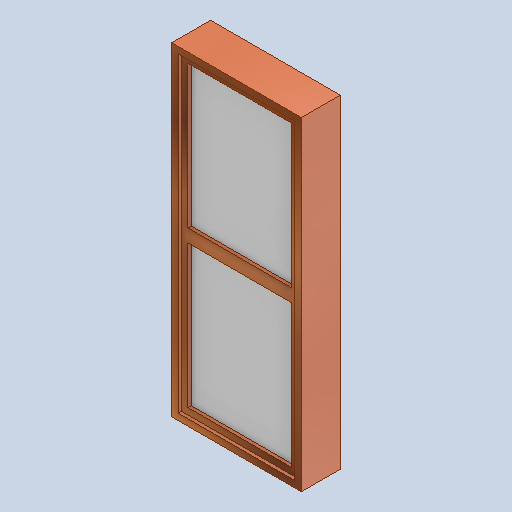
# Autodesk Inventor part: 窗_無底
Saved by Autodesk Inventor 2024.2 (Build 282272000, 272)
## iProperties
Created: 2024-05-31
Part Number: 窗_無底
Material: 木材 (胡桃木)
Document SubType Name: Modeling
Designer: User
Density: 0.55 g/cm^3
Appearance: 胡桃木 - 天然拋光
Author: User
Autodesk Inventor part; units mm, degrees
ref_plane "YZ Plane" through (0, 0, 0) normal (1, 0, 0) x (0, 1, 0)
ref_plane "XZ Plane" through (0, 0, 0) normal (0, 1, 0) x (-1, 0, 0)
ref_plane "XY Plane" through (0, 0, 0) normal (0, 0, 1) x (1, 0, 0)
sketch "草圖1" plane through (0, 0, 0) normal (0, 0, 1) x (1, 0, 0)
  line L0 (-1, 2.5) -> (1, 2.5)
  line L1 (1, 2.5) -> (1, -2.5)
  line L2 (1, -2.5) -> (-1, -2.5)
  line L3 (-1, -2.5) -> (-1, 2.5)
  line L4 (-1, 2.5) -> (1, -2.5) construction
  line L5 (1, 2.5) -> (-1, -2.5) construction
  line L6 (-0.8, -0.1) -> (0.8, -0.1)
  line L7 (1, -0.1) -> (1, 0.1)
  line L8 (0.8, 0.1) -> (-0.8, 0.1)
  line L9 (-1, 0.1) -> (-1, -0.1)
  line L10 (-1, -0.1) -> (1, 0.1) construction
  line L11 (1, -0.1) -> (-1, 0.1) construction
  line L12 (-0.8, -2.3) -> (0.8, -2.3)
  line L13 (0.8, 2.3) -> (-0.8, 2.3)
  line L14 (-0.8, 2.3) -> (0.8, -2.3) construction
  line L15 (-0.8, -2.3) -> (0.8, 2.3) construction
  line L16 (0.8, -2.3) -> (0.8, -0.08)
  line L17 (0.8, 0.08) -> (0.8, 2.3)
  line L18 (-0.8, 2.3) -> (-0.8, 0.08)
  line L19 (-0.8, -0.08) -> (-0.8, -2.3)
  line L20 (-1, -2.5) -> (1, -2.5)
  line L21 (1, -2.5) -> (1, -5.5)
  line L22 (1, -5.5) -> (-1, -5.5)
  line L23 (-1, -5.5) -> (-1, -2.5)
  line L24 (-0.9, -2.4) -> (0.9, -2.4)
  line L25 (0.9, -2.4) -> (0.9, 2.4)
  line L26 (0.9, 2.4) -> (-0.9, 2.4)
  line L27 (-0.9, 2.4) -> (-0.9, -2.4)
  line L28 (-0.9, -2.4) -> (0.9, 2.4) construction
  line L29 (0.9, -2.4) -> (-0.9, 2.4) construction
  point P0 (0, 0)
  dimension "d0" = 2
  dimension "d1" = 5
  dimension "d4" = 0.2
  dimension "d5" = 4.6
  dimension "d6" = 1.6
  dimension "d7" = 3
  dimension "d12" = 1.8
  dimension "d13" = 4.8
  constraints: 60 end point, 14 equal length, 8 midpoint, 8 perpendicular, 8 point on line, 2 horizontal
  measures "d0" distance of L0.start L0.end
  measures "d1" distance of L0.end L1.end
  measures "d4" distance of L7.end L7.start
  measures "d5" distance of L13.end L12.start
  measures "d6" distance of L12.end L12.start
  measures "d7" distance of L1.end L21.end
  measures "d12" distance of L24.start L24.end
  measures "d13" distance of L25.end L24.end
extrude "擠出4" add sketch "草圖1" along normal blind 0.6 contours L0 L1 L2 L3
extrude "擠出5" add sketch "草圖1" along normal blind 0.55 contours L27 L26 L25 L24
extrude "擠出6" add sketch "草圖1" along normal blind 0.5 contours L2 L21 L22 L23 | L6 L16 L12 L19 | L8 L18 L13 L17
sketch "草圖3" plane through (-1, -2.5, 0.6) normal (-1, 0, 0) x (0, 0, 1)
  line L0 (-0.6, 5) -> (-0.6, -3) projected
  line L1 (-0.6, -3) -> (-0.1, -3) projected
  line L2 (-0.1, 0) -> (-0.1, -3) projected
  line L3 (-0.1, 0) -> (0, 0) projected
  line L4 (0, 5) -> (0, 0) projected
  line L5 (-0.6, 5) -> (0, 5) projected
  line L6 (-0.6, 0) -> (-0.1, 0)
  line L7 (-0.1, 0) -> (-0.1, -3)
  line L8 (-0.1, -3) -> (-0.6, -3)
  line L9 (-0.6, -3) -> (-0.6, 0)
  point P0 (-0.6, 2.5)
  constraints: 8 end point, 2 parallel, 2 perpendicular, 1 point on line
extrude "擠出8" cut sketch "草圖3" against normal blind 2 contours L6 L2 L1 L0
